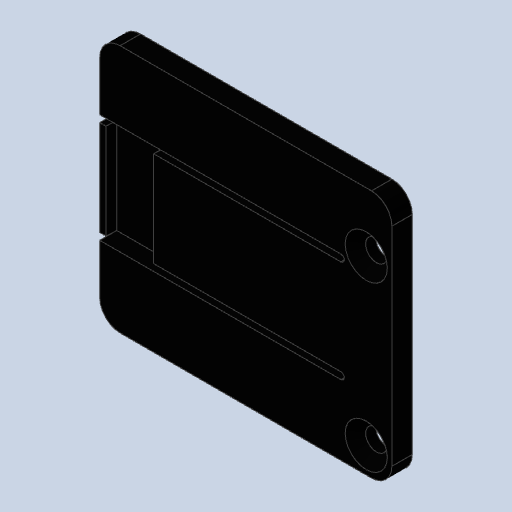
# Autodesk Inventor part: test_akkum_shelki
Saved by Autodesk Inventor 2022 (Build 260153000, 153)
## iProperties
Created: 2022-12-06
Part Number: test_akkum_shelki
Material: Generic
Document SubType Name: Modeling
Designer: akapu
Density: 1 g/cm^3
Appearance: Default
Author: akapu
Autodesk Inventor part; units mm, degrees
ref_plane "YZ Plane" through (0, 0, 0) normal (1, 0, 0) x (0, 1, 0)
ref_plane "XZ Plane" through (0, 0, 0) normal (0, 1, 0) x (-1, 0, 0)
ref_plane "XY Plane" through (0, 0, 0) normal (0, 0, 1) x (1, 0, 0)
sketch "Sketch1" plane through (0, 0, 0) normal (0, 0, 1) x (1, 0, 0)
  circle A0 centre (17.7236, 9.6) radius 1.6 projected
  circle A1 centre (17.7236, -14.5236) radius 1.6 projected
  line L0 (7.5226, -3.6515) -> (7.5226, 2.8) projected
  line L1 (7.5226, -3.6515) -> (9.3355, -5.4645) projected
  arc A2 (1.9766, -12.2221) -> (9.3355, -5.4645) centre (5.8, -9) ccw projected
  spline S0 degree 2 poles (1.9766, -12.2221) (-3.2, -10.4641) (-8.3766, -12.2221) knots 0.21241 0.21241 0.21241 0.78759 0.78759 0.78759 projected
  arc A3 (-15.4221, -5.1766) -> (-8.3766, -12.2221) centre (-12.2, -9) ccw projected
  spline S1 degree 2 poles (-15.4221, -5.1766) (-13.6641, 0) (-15.4221, 5.1766) knots 0.212408 0.212408 0.212408 0.787591 0.787591 0.787591 projected
  arc A4 (-8.6645, 12.5355) -> (-15.4221, 5.1766) centre (-12.2, 9) ccw projected
  line L2 (-8.6645, 12.5355) -> (-5.3142, 9.1853) projected
  arc A5 (-5.3142, 9.1853) -> (-2.6505, 9.0378) centre (-3.9, 10.5995) ccw projected
  arc A6 (-2.6505, 9.0378) -> (-2.5046, 9) centre (-2.5046, 9.3) ccw projected
  line L3 (-2.5046, 9) -> (-1.9, 9) projected
  arc A7 (3.1749, 12.6) -> (-1.9, 9) centre (7.9405, 0.505) ccw projected
  line L4 (3.1749, 12.6) -> (15.5327, 12.6) projected
  arc A8 (15.7904, 11.8941) -> (15.5327, 12.6) centre (15.5327, 12.2) ccw projected
  arc A9 (15.7904, 11.8941) -> (17.7236, 6.6) centre (17.7236, 9.6) ccw projected
  line L5 (18.5, 6.6) -> (17.7236, 6.6) projected
  line L6 (18.5, 6.6) -> (18.5, 2.8) projected
  line L7 (7.5226, 2.8) -> (18.5, 2.8) projected
  line L8 (-18.5, -18.3) -> (18.5, -18.3) projected
  arc A10 (18.5, -18.3) -> (21.5, -15.3) centre (18.5, -15.3) ccw projected
  line L9 (21.5, -15.3) -> (21.5, 15.3) projected
  arc A11 (21.5, 15.3) -> (18.5, 18.3) centre (18.5, 15.3) ccw projected
  line L10 (18.5, 18.3) -> (-18.5, 18.3) projected
  arc A12 (-18.5, 18.3) -> (-21.5, 15.3) centre (-18.5, 15.3) ccw projected
  line L11 (-21.5, 15.3) -> (-21.5, -15.3) projected
  arc A13 (-21.5, -15.3) -> (-18.5, -18.3) centre (-18.5, -15.3) ccw projected
  line L12 (-21.5, 0) -> (-21.5, -8)
  line L13 (-21.5, -8) -> (-21.5, -7)
  line L14 (-21.5, -7) -> (21.5, -7)
  line L15 (-21.5, -8) -> (21.5, -8)
  line L16 (-21.5, -7) -> (14.5, -7)
  line L17 (14.5, -8) -> (14.5, 0)
  line L18 (14.5, 0) -> (-21.5, 0)
  line L19 (-21.5, -15.3) -> (-21.5, 15.3)
  line L20 (-21.5, 7) -> (21.5, 7)
  line L21 (-21.5, 8) -> (21.5, 8)
  line L22 (14.5, 8) -> (14.5, 0)
  point P0 (0, 0)
  point P1 (10.699, -8)
  point P2 (14.5, 7)
  point P3 (10.3826, -7)
  dimension "d0" = 8
  dimension "d1" = 1
  dimension "d2" = 36
  constraints: 22 end point, 8 point on line, 7 symmetric about line, 3 perpendicular, 1 horizontal, 1 midpoint
  measures "d0" distance of L12.start L12.end
  measures "d1" distance of L12.end L13.end
  measures "d2" distance of L13.end L16.end
extrude "Extrusion1" add sketch "Sketch1" along normal blind 3 contours L21 A9 A8 L4 A7 L3 A6 A5 L2 A4 L11 A12 L10 A11 L9 | L21 L9 L20 A9 | L21 A4 L2 A5 A6 L3 A7 L4 A8 A9 | A9 L20 L22 L21 | L20 L9 L14 L17 L22 L7 L6 L5 A9 | A9 L5 L6 L7 L22 L20 | L22 L7 L0 L18 S1 A4 L20 | L9 L15 L17 L14 | A4 S1 L18 L11 L20 | L22 L18 L0 L7 | L9 A10 L8 A13 L11 L15 A3 S0 A2 | L14 A2 L1 L0 L18 L17 | L14 A3 S1 L18 L0 L1 A2 | S1 A3 L14 L11 L18 | A2 S0 A3 L15
chamfer "Chamfer1" distance 1.5 angle 45 2 edges at (16.1236, -14.5236, 3) (16.1236, 9.6, 3)
sketch "Sketch2" plane through (-21.5, 7, 0) normal (0, 1, 0) x (1, 0, 0)
  line L0 (36, 0) -> (36, -3) projected
  line L1 (36, 0) -> (36, -3)
  line L2 (0, -3) -> (3, -3) projected
  line L3 (36, 0) -> (0, 0)
  line L4 (0, 0) -> (0, -3)
  line L5 (0, -3) -> (36, -3)
  line L6 (36, -3) -> (36, 0)
  line L7 (0, -3) -> (7.914, -3)
  line L8 (3, -3) -> (40, -3) projected
  line L9 (0, 0) -> (0, -3) projected
  line L10 (0, -1.5) -> (8, -1.5)
  line L11 (8, -1.5) -> (7.914, -3)
  line L12 (0, 0) -> (10, 0)
  line L13 (0, 0) -> (36, 0) projected
  line L14 (10, 0) -> (36, -1.5)
  line L15 (0, -1.5) -> (1, -1.5)
  line L16 (1, -1.5) -> (0.914, -3)
  line L17 (0, -3) -> (36, -3) projected
  point P0 (21.5, 0)
  point P1 (7.914, -3)
  point P2 (0, -1.5)
  point P3 (0.914, -3)
  dimension "d8" = 7.914
  dimension "d9" = 8
  dimension "d10" = 10
  dimension "d14" = 1
  constraints: 24 end point, 4 point on line, 3 equal length, 2 horizontal, 2 midpoint, 1 perpendicular
  measures "d8" distance of L2.start L7.end
  measures "d9" distance of L10.start L10.end
  measures "d10" distance of L3.end L12.end
  measures "d14" distance of L10.start L15.end
extrude "Extrusion2" cut sketch "Sketch2" against normal up to surface (14 mm away) contours L0 L14 L3 | L5 L2 L16 L10 L11
fillet "Fillet1" radius 0.5 4 edges at (14.5, 8, 1.5) (14.5, 7, 2.25) (14.5, -7, 2.25) (14.5, -8, 1.5)
body "Solid1"
